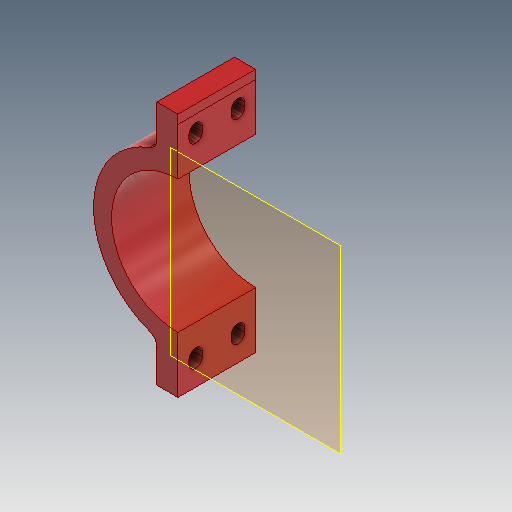
# Autodesk Inventor part: motor mount cap
Saved by Autodesk Inventor 2020 (Build 240168000, 168)
## iProperties
Created: 2019-10-28
Part Number: motor mount cap
Material: Generic
Document SubType Name: Modeling
Designer: ball
Density: 1 g/cm^3
Appearance: Default
Author: ball
Autodesk Inventor part; units mm, degrees
ref_plane "YZ Plane" through (0, 0, 0) normal (1, 0, 0) x (0, 1, 0)
ref_plane "XZ Plane" through (0, 0, 0) normal (0, 1, 0) x (-1, 0, 0)
ref_plane "Work Plane1" through (0, 0, 0) normal (0, 0, 1) x (1, 0, 0)
sketch "Sketch1" plane through (0, 0, 0) normal (0, 0, 1) x (1, 0, 0)
  arc A0 (18.9992, 41.108) -> (0, 60.0877) centre (-0.0008, 41.0877) ccw construction
  arc A1 (0, 22.1284) -> (18.9992, 41.108) centre (-0.0008, 41.1284) ccw construction
  arc A2 (44.3468, 60.0877) -> (25.3476, 41.108) centre (44.3476, 41.0877) ccw construction
  arc A3 (25.3476, 41.108) -> (44.3468, 22.1284) centre (44.3476, 41.1284) ccw construction
  line L0 (10.16, 73.6386) -> (5.7912, 73.6386) construction
  line L1 (0, 77.677) -> (0, 67.7202) construction
  line L2 (5.7912, 73.6386) -> (13.9012, 73.6386) construction
  line L3 (-25.35, 77.677) -> (-25.35, 84.027) projected
  line L4 (-25.35, -6.35) -> (-25.35, 0) projected
  line L5 (-25.35, 77.677) -> (-25.35, 0) construction
  arc A4 (-6.0324, 64.4924) -> (-6.0325, 17.7644) centre (-0.0008, 41.1284) ccw
  arc A5 (-6.0324, 64.4924) -> (-6.0325, 17.7644) centre (-0.0008, 41.1284) ccw
  arc A6 (-0.0008, 60.1276) -> (-0.0008, 22.1292) centre (-0.0008, 41.1284) ccw
  line L6 (-6.0324, 64.4924) -> (-6.0324, 73.6793)
  line L7 (10.16, 8.5775) -> (5.7912, 8.5775) construction
  line L8 (-6.0325, 8.5775) -> (-6.0325, 17.7644)
  line L9 (-0.0008, 73.6793) -> (-0.0008, 60.1276)
  line L10 (-0.0008, 8.5775) -> (-0.0008, 22.1292)
  line L11 (-6.0324, 73.6793) -> (-6.0324, 76.2193)
  line L12 (-6.0324, 76.2193) -> (0, 76.2193)
  line L13 (-0.0008, 73.6793) -> (0, 76.2193)
  line L14 (-6.0325, 8.5775) -> (-6.0325, 6.0375)
  line L15 (-6.0325, 6.0375) -> (-0.0008, 6.0375)
  line L16 (-0.0008, 6.0375) -> (-0.0008, 8.5775)
  point P0 (0, 0)
  dimension "d12" = 18.9992
  dimension "d13" = 24.13
  dimension "d19" = 6.0317
  dimension "d22" = 6.0317
  dimension "d23" = 0
  dimension "d24" = 0
  dimension "d44" = 2.54
  dimension "d45" = 2.54
  constraints: 24 end point, 7 point on circle, 5 vertical, 3 centre point, 2 perpendicular, 2 point on line, 1 coincident, 1 horizontal
  measures "d12" radius of A6
  measures "d13" radius of A5
  measures "d19" distance from line of L8 A1.centre
  measures "d22" distance from line of L6 A0.centre
  measures "d23" distance from line of L9 A0.centre
  measures "d24" distance from line of L10 A0.centre
  measures "d44" distance of L6.end L11.end
  measures "d45" distance of L8.start L14.end
ref_plane "Work Plane2" through (0, 17.6708, -22.228) normal (0, 0, -1) x (0, 1, 0)
extrude "Extrusion1" add sketch "Sketch1" against normal up to surface (22.228 mm away)
fillet "Fillet1" radius 3.175 1 edges at (-6.0324, 64.4924, -11.114)
fillet "Fillet2" radius 3.175 1 edges at (-6.0325, 17.7644, -11.114)
sketch "Sketch3" plane through (-6.0325, 8.5775, -22.228) normal (-1, 0, 0) x (0, 0, 1)
  circle A0 centre (5.08, 4.7016) radius 1.9304 construction
  circle A1 centre (17.148, 4.7016) radius 1.9304 construction
  circle A2 centre (17.148, 60.4409) radius 1.9304 construction
  circle A3 centre (5.08, 60.4409) radius 1.9304 construction
  line L0 (5.08, 4.0666) -> (5.08, 5.3366) construction
  line L1 (7.0104, 4.0666) -> (7.0104, 5.3366)
  line L2 (3.1496, 5.3366) -> (3.1496, 4.0666)
  arc A4 (3.1496, 4.0666) -> (7.0104, 4.0666) centre (5.08, 4.0666) ccw
  arc A5 (7.0104, 5.3366) -> (3.1496, 5.3366) centre (5.08, 5.3366) ccw
  point P0 (22.228, -8.5775)
  point P1 (5.08, 7.9375)
  dimension "d25" = 0.635
  dimension "d26" = 0.635
  dimension "d27" = 3.8608
  constraints: 8 end point, 4 point on circle, 4 tangent, 2 centre point, 1 coincident, 1 midpoint, 1 parallel, 1 vertical
  measures "d25" distance of L0.start point (5.08, 4.702)
  measures "d26" distance of L0.end point (5.08, 4.702)
  measures "d27" diameter of A5
extrude "Extrusion3" cut sketch "Sketch3" against normal through all both and the other way through all
sketch "Sketch4" plane through (-6.0325, 8.5775, -22.228) normal (-1, 0, 0) x (0, 0, 1)
  circle A0 centre (17.148, 4.7016) radius 1.9304 construction
  circle A1 centre (5.08, 60.4409) radius 1.9304 construction
  circle A2 centre (17.148, 60.4409) radius 1.9304 construction
  line L0 (17.148, 4.0666) -> (17.148, 5.3366) construction
  line L1 (19.0784, 4.0666) -> (19.0784, 5.3366)
  line L2 (15.2176, 5.3366) -> (15.2176, 4.0666)
  arc A3 (15.2176, 4.0666) -> (19.0784, 4.0666) centre (17.148, 4.0666) ccw
  arc A4 (19.0784, 5.3366) -> (15.2176, 5.3366) centre (17.148, 5.3366) ccw
  line L3 (5.08, 59.8059) -> (5.08, 61.0759) construction
  line L4 (7.0104, 59.8059) -> (7.0104, 61.0759)
  line L5 (3.1496, 61.0759) -> (3.1496, 59.8059)
  arc A5 (3.1496, 59.8059) -> (7.0104, 59.8059) centre (5.08, 59.8059) ccw
  arc A6 (7.0104, 61.0759) -> (3.1496, 61.0759) centre (5.08, 61.0759) ccw
  line L6 (17.148, 59.8059) -> (17.148, 61.0759) construction
  line L7 (19.0784, 59.8059) -> (19.0784, 61.0759)
  line L8 (15.2176, 61.0759) -> (15.2176, 59.8059)
  arc A7 (15.2176, 59.8059) -> (19.0784, 59.8059) centre (17.148, 59.8059) ccw
  arc A8 (19.0784, 61.0759) -> (15.2176, 61.0759) centre (17.148, 61.0759) ccw
  point P0 (22.228, -8.5775)
  point P1 (17.148, 4.7016)
  dimension "d30" = 0.635
  dimension "d31" = 0.635
  dimension "d32" = 0.635
  dimension "d33" = 0.635
  dimension "d34" = 0.635
  dimension "d35" = 0.635
  dimension "d36" = 3.8608
  dimension "d37" = 3.8608
  dimension "d38" = 3.8608
  constraints: 24 end point, 12 point on circle, 12 tangent, 6 centre point, 5 parallel, 3 midpoint, 1 vertical
  measures "d30" distance of L0.end A0.centre
  measures "d31" distance of L0.start A0.centre
  measures "d32" distance of L3.start A1.centre
  measures "d33" distance of A1.centre L3.end
  measures "d34" distance of L6.start A2.centre
  measures "d35" distance of A2.centre L6.end
  measures "d36" diameter of A4
  measures "d37" diameter of A6
  measures "d38" diameter of A8
extrude "Extrusion4" cut sketch "Sketch4" against normal through all both and the other way through all
equation "\"d19\" = d18"
equation "\"d18\" = 6.031656"
body "Solid1"
